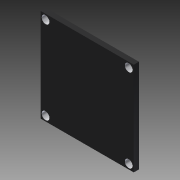
# Autodesk Inventor part: PDB 36x36
Saved by Autodesk Inventor 2015 (Build 190159000, 159)
## iProperties
Created: 2016-11-27
Part Number: PDB 36x36
Material: Generic
Document SubType Name: Modeling
Designer: Hampus
Density: 1 g/cm^3
Appearance: Rubber - Black
Author: Hampus
Autodesk Inventor part; units mm, degrees
ref_plane "YZ Plane" through (0, 0, 0) normal (1, 0, 0) x (0, 1, 0)
ref_plane "XZ Plane" through (0, 0, 0) normal (0, 1, 0) x (-1, 0, 0)
ref_plane "XY Plane" through (0, 0, 0) normal (0, 0, 1) x (1, 0, 0)
sketch "Sketch1" plane through (0, 0, 0) normal (0, 1, 0) x (-1, 0, 0)
  line L0 (0, 0) -> (-36, 0)
  line L1 (-36, 0) -> (-36, -36)
  line L2 (-36, -36) -> (0, -36)
  line L3 (0, -36) -> (0, 0)
  circle A0 centre (-1.9445, -34.0555) radius 1.5
  circle A1 centre (-34.0555, -34.0555) radius 1.5
  circle A2 centre (-1.9445, -1.9445) radius 1.5
  circle A3 centre (-34.0555, -1.9445) radius 1.5
  line L4 (-6.1012, -34.6884) -> (-8.9666, -34.6884)
  line L5 (-8.9666, -34.6884) -> (-8.9666, -32.1278)
  line L6 (-8.9666, -32.1278) -> (-6.1012, -32.1278)
  line L7 (-6.1012, -32.1278) -> (-6.1012, -34.6884)
  line L8 (-11.5272, -34.6884) -> (-14.4536, -34.6884)
  line L9 (-14.4536, -34.6884) -> (-14.4536, -32.1278)
  line L10 (-14.4536, -32.1278) -> (-11.5272, -32.1278)
  line L11 (-11.5272, -32.1278) -> (-11.5272, -34.6884)
  line L12 (-17.5019, -34.6884) -> (-20.6111, -34.6884)
  line L13 (-20.6111, -34.6884) -> (-20.6111, -32.1278)
  line L14 (-20.6111, -32.1278) -> (-17.5019, -32.1278)
  line L15 (-17.5019, -32.1278) -> (-17.5019, -34.6884)
  line L16 (-23.9642, -34.6884) -> (-27.6831, -34.6884)
  line L17 (-27.6831, -34.6884) -> (-27.6831, -32.1278)
  line L18 (-27.6831, -32.1278) -> (-23.9642, -32.1278)
  line L19 (-23.9642, -32.1278) -> (-23.9642, -34.6884)
  line L20 (-34.6332, -30.055) -> (-31.9508, -30.055)
  line L21 (-31.9508, -30.055) -> (-31.9508, -27.5554)
  line L22 (-31.9508, -27.5554) -> (-34.6332, -27.5554)
  line L23 (-34.6332, -27.5554) -> (-34.6332, -30.055)
  line L24 (-34.6332, -24.0803) -> (-31.585, -24.0803)
  line L25 (-31.585, -24.0803) -> (-31.585, -21.9465)
  line L26 (-31.585, -21.9465) -> (-34.6332, -21.9465)
  line L27 (-34.6332, -21.9465) -> (-34.6332, -24.0803)
  line L28 (-34.6332, -18.8373) -> (-31.585, -18.8373)
  line L29 (-31.585, -18.8373) -> (-31.585, -16.2767)
  line L30 (-31.585, -16.2767) -> (-34.6332, -16.2767)
  line L31 (-34.6332, -16.2767) -> (-34.6332, -18.8373)
  line L32 (-34.0555, -11.8872) -> (-31.585, -11.8872)
  line L33 (-31.585, -11.8872) -> (-31.585, -7.6196)
  line L34 (-31.585, -7.6196) -> (-34.0555, -7.6196)
  line L35 (-34.0555, -7.6196) -> (-34.0555, -11.8872)
  line L36 (-28.7805, -2.6813) -> (-25.4884, -2.6813)
  line L37 (-25.4884, -2.6813) -> (-25.4884, -0.4445)
  line L38 (-25.4884, -0.4445) -> (-28.7805, -0.4445)
  line L39 (-28.7805, -0.4445) -> (-28.7805, -2.6813)
  line L40 (-21.0379, -2.6813) -> (-16.2825, -2.6813)
  line L41 (-16.2825, -2.6813) -> (-16.2825, -0.4445)
  line L42 (-16.2825, -0.4445) -> (-21.0379, -0.4445)
  line L43 (-21.0379, -0.4445) -> (-21.0379, -2.6813)
  line L44 (-13.661, -3.4445) -> (-10.4298, -3.4445)
  line L45 (-10.4298, -3.4445) -> (-10.4298, -1.0962)
  line L46 (-10.4298, -1.0962) -> (-13.661, -1.0962)
  line L47 (-13.661, -1.0962) -> (-13.661, -3.4445)
  line L48 (-6.1012, -3.4445) -> (-4.2113, -3.4445)
  line L49 (-4.2113, -3.4445) -> (-4.2113, -0.4445)
  line L50 (-4.2113, -0.4445) -> (-6.1012, -0.4445)
  line L51 (-6.1012, -0.4445) -> (-6.1012, -3.4445)
  line L52 (-2.4433, -7.6196) -> (-0.4445, -7.6196)
  line L53 (-0.4445, -7.6196) -> (-0.4445, -5.12)
  line L54 (-0.4445, -5.12) -> (-2.4433, -5.12)
  line L55 (-2.4433, -5.12) -> (-2.4433, -7.6196)
  line L56 (-2.4433, -13.5942) -> (-0.8582, -13.5942)
  line L57 (-0.8582, -13.5942) -> (-0.8582, -10.363)
  line L58 (-0.8582, -10.363) -> (-2.4433, -10.363)
  line L59 (-2.4433, -10.363) -> (-2.4433, -13.5942)
  line L60 (-3.4445, -19.6298) -> (-0.8582, -19.6298)
  line L61 (-0.8582, -19.6298) -> (-0.8582, -15.5451)
  line L62 (-0.8582, -15.5451) -> (-3.4445, -15.5451)
  line L63 (-3.4445, -15.5451) -> (-3.4445, -19.6298)
  line L64 (-2.931, -25.9703) -> (-0.8582, -25.9703)
  line L65 (-0.8582, -25.9703) -> (-0.8582, -22.6781)
  line L66 (-0.8582, -22.6781) -> (-2.931, -22.6781)
  line L67 (-2.931, -22.6781) -> (-2.931, -25.9703)
  line L68 (-2.931, -30.6646) -> (-0.8582, -30.6646)
  line L69 (-0.8582, -30.6646) -> (-0.8582, -28.8052)
  line L70 (-0.8582, -28.8052) -> (-2.931, -28.8052)
  line L71 (-2.931, -28.8052) -> (-2.931, -30.6646)
  line L72 (-27.6831, -30.055) -> (-6.528, -30.055)
  line L73 (-6.528, -30.055) -> (-6.528, -25.9703)
  line L74 (-6.528, -25.9703) -> (-27.6831, -25.9703)
  line L75 (-27.6831, -25.9703) -> (-27.6831, -30.055)
  line L76 (-6.528, -23.5926) -> (-27.6831, -23.5926)
  line L77 (-27.6831, -23.5926) -> (-27.6831, -18.8373)
  line L78 (-27.6831, -18.8373) -> (-6.528, -18.8373)
  line L79 (-6.528, -18.8373) -> (-6.528, -23.5926)
  line L80 (-25.8237, -9.2047) -> (-8.5399, -9.2047)
  line L81 (-8.5399, -9.2047) -> (-8.5399, -16.2767)
  line L82 (-8.5399, -16.2767) -> (-25.8237, -16.2767)
  line L83 (-25.8237, -16.2767) -> (-25.8237, -9.2047)
  dimension "d2" = 3
  dimension "d3" = 3
  constraints: 168 end point, 42 parallel, 28 point on line, 21 horizontal, 21 perpendicular, 4 centre point
  measures "d2" diameter of A0
  measures "d3" diameter of A1
extrude "Extrusion1" add sketch "Sketch1" along normal blind 2 contours L3 L2 L1 L0 | L4 L5 L6 L7 | L8 L9 L10 L11 | L12 L13 L14 L15 | L16 L17 L18 L19 | L23 L22 L21 L20 | L27 L26 L25 L24 | L31 L30 L29 L28 | L35 L34 L33 L32 | L39 L38 L37 L36 | L43 L42 L41 L40 | L47 L46 L45 L44 | L51 L50 L49 L48 | L55 L54 L53 L52 | L59 L58 L57 L56 | L63 L62 L61 L60 | L67 L66 L65 L64 | L71 L70 L69 L68 | L75 L74 L73 L72 | L76 L77 L78 L79 | L80 L81 L82 L83
extrude "Extrusion2" add sketch "Sketch1" along normal blind 2.2 contours L4 L5 L6 L7 | L8 L9 L10 L11 | L12 L13 L14 L15 | L16 L17 L18 L19 | L23 L22 L21 L20 | L27 L26 L25 L24 | L31 L30 L29 L28 | L35 L34 L33 L32 | L39 L38 L37 L36 | L43 L42 L41 L40 | L47 L46 L45 L44 | L51 L50 L49 L48 | L55 L54 L53 L52 | L59 L58 L57 L56 | L63 L62 L61 L60 | L67 L66 L65 L64 | L71 L70 L69 L68 | L75 L74 L73 L72 | L76 L77 L78 L79 | L80 L81 L82 L83
body "Solid1"
